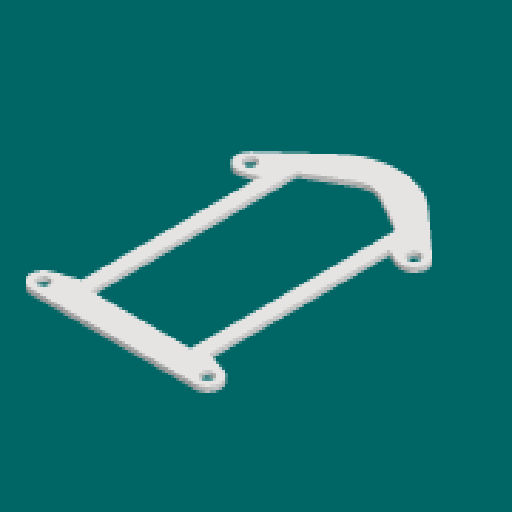
# Autodesk Inventor part: Skirt
Saved by Autodesk Inventor 2023 (Build 270158000, 158)
## iProperties
Created: 2022-10-14
Part Number: Skirt
Material: 一般
Document SubType Name: Modeling
Designer: hide
Density: 1 g/cm^3
Appearance: 既定
Author: hide
Autodesk Inventor part; units mm, degrees
ref_plane "YZ Plane" through (0, 0, 0) normal (1, 0, 0) x (0, 1, 0)
ref_plane "XZ Plane" through (0, 0, 0) normal (0, 1, 0) x (-1, 0, 0)
ref_plane "XY Plane" through (0, 0, 0) normal (0, 0, 1) x (1, 0, 0)
sketch "スケッチ1" plane through (0, 0, 0) normal (0, 1, 0) x (-1, 0, 0)
  circle A0 centre (11.5, 0) radius 0.85
  circle A1 centre (11.5, 29) radius 0.85
  line L0 (0, -11.6446) -> (0, 36.0381)
  line L1 (10.8673, 1.7384) -> (9, 1.0588)
  line L2 (9, 1.0588) -> (9, 26.1213)
  line L3 (9, 26.1213) -> (12.1327, 27.2616)
  arc A2 (12.1327, 27.2616) -> (11.5, 30.85) centre (11.5, 29) ccw
  arc A3 (12.5698, -1.5093) -> (10.8673, 1.7384) centre (11.5, 0) ccw
  circle A4 centre (0, 0) radius 7.5
  line L4 (11.5, 30.85) -> (0, 30.85)
  line L5 (0, 26.85) -> (7, 26.85)
  line L6 (7, 26.85) -> (7, 2.6926)
  line L7 (7, 2.6926) -> (2.9803, -3.8352)
  circle A5 centre (-11.5, 0) radius 0.85
  circle A6 centre (-11.5, 29) radius 0.85
  line L8 (-10.8673, 1.7384) -> (-9, 1.0588)
  line L9 (-9, 1.0588) -> (-9, 26.1213)
  line L10 (-9, 26.1213) -> (-12.1327, 27.2616)
  arc A7 (-11.5, 30.85) -> (-12.1327, 27.2616) centre (-11.5, 29) ccw
  arc A8 (-10.8673, 1.7384) -> (-12.5698, -1.5093) centre (-11.5, 0) ccw
  line L11 (-11.5, 30.85) -> (0, 30.85)
  line L12 (0, 26.85) -> (-7, 26.85)
  line L13 (-7, 26.85) -> (-7, 2.6926)
  line L14 (-7, 2.6926) -> (-2.9803, -3.8352)
  line L15 (12.5698, -1.5093) -> (4.9152, -6.9347)
  arc A9 (0, -8.5) -> (4.9152, -6.9347) centre (0, 0) ccw
  line L16 (-12.5698, -1.5093) -> (-4.9152, -6.9347)
  arc A10 (-4.9152, -6.9347) -> (0, -8.5) centre (0, 0) ccw
  circle A11 centre (0, -2) radius 3.5
  point P0 (7, 2.6926)
  point P1 (-7, 2.6926)
  point P2 (-2.9803, -3.8352)
  dimension "d7" = 15
  dimension "d23" = 7
  dimension "d2" = 29
  dimension "d4" = 23
  dimension "d10" = 1
  dimension "d11" = 1
  dimension "d12" = 18
  dimension "d13" = 2
  dimension "d14" = 4
  dimension "d18" = 8.5
  dimension "d19" = 20
  dimension "d24" = 1.7
  dimension "d25" = 2
  constraints: 34 end point, 14 symmetric about line, 12 point on circle, 10 centre point, 6 coincident, 5 point on line, 5 tangent, 2 perpendicular, 2 vertical, 1 equal radius, 1 horizontal, 1 horizontal alignment, 1 parallel, 1 vertical alignment, 12 other
  measures "d2" distance of A1.centre A0.centre
  measures "d4" diameter of A0.centre L0
  measures "d10" radial gap between concentric circles of A3 A0
  measures "d11" radial gap between concentric circles of A2 A1
  measures "d12" diameter of L2 L0
  measures "d13" distance between parallel lines of L2 L6
  measures "d14" distance between parallel lines of L4 L5
  measures "d18" radius of A9
  measures "d19" angle of L4 L3
  measures "d24" diameter of A0
  measures "d25" distance of point (0, 0) point (0, -2)
extrude "押し出し1" add sketch "スケッチ1" along normal blind 0.7 contours L12 L13 A4 L0 A10 L16 A8 L8 L9 L10 A7 L11 | L0 L4 A2 L3 L2 L1 A3 L15 A9 A4 L6 L5 | A4 L0 A11 L7 | L14 A11 L0 A4 picked at (5.9308, -1.8347) picked at (-5.8073, -0.0693)
